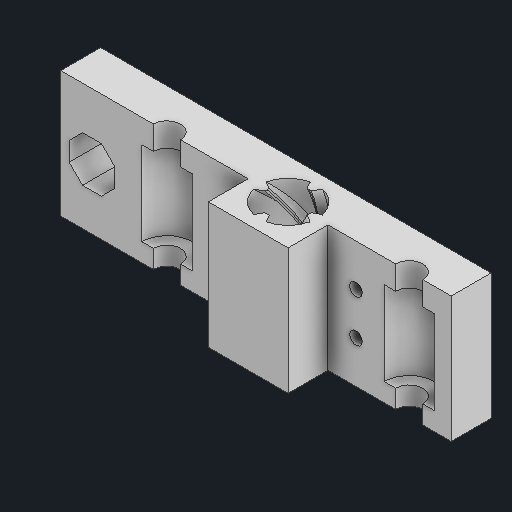
# Autodesk Inventor part: carriage_slider_bottom
Saved by Autodesk Inventor 2025 (Build 290162010, 162A)
## iProperties
Created: 2024-06-23
Part Number: carriage_slider_bottom
Material: Generic
Document SubType Name: Modeling
Designer: mihir
Density: 1 g/cm^3
Appearance: Default
Author: mihir
Autodesk Inventor part; units mm, degrees
ref_plane "YZ Plane" through (0, 0, 0) normal (1, 0, 0) x (0, 1, 0)
ref_plane "XZ Plane" through (0, 0, 0) normal (0, 1, 0) x (-1, 0, 0)
ref_plane "XY Plane" through (0, 0, 0) normal (0, 0, 1) x (1, 0, 0)
sketch "Sketch1" plane through (0, 0, 0) normal (0, 1, 0) x (-1, 0, 0)
  line L0 (-9.5, 9.5) -> (9.5, 9.5)
  line L1 (9.5, 9.5) -> (9.5, -9.5)
  line L2 (9.5, -9.5) -> (-9.5, -9.5)
  line L3 (-9.5, -9.5) -> (-9.5, 9.5)
  line L4 (-9.5, 9.5) -> (9.5, -9.5) construction
  line L5 (9.5, 9.5) -> (-9.5, -9.5) construction
  circle A0 centre (0, 0) radius 6.875
  dimension "d0" = 13.75
  dimension "d1" = 9.5
  constraints: 12 end point, 2 midpoint, 2 parallel, 2 perpendicular, 1 centre point, 1 coincident, 1 horizontal
  measures "d0" diameter of A0
  measures "d1" distance from line of L1 A0.centre
extrude "Extrusion1" add sketch "Sketch1" along normal blind 30
sketch "Sketch2" plane through (0, 30, 0) normal (0, 1, 0) x (1, 0, 0)
  circle A0 centre (0, 0) radius 5 construction
  circle A1 centre (0, 0) radius 6.875 projected
  line L0 (0, -6.875) -> (-1.5825, -6.875)
  line L1 (-1.5825, -6.875) -> (-0.5, -5)
  line L2 (-0.5, -5) -> (0, -5)
  line L3 (0, -6.875) -> (0, -5)
  line L4 (0, -5) -> (0, 0) construction
  line L5 (0, -6.875) -> (1.5825, -6.875)
  line L6 (1.5825, -6.875) -> (0.5, -5)
  line L7 (0.5, -5) -> (0, -5)
  dimension "d4" = 10
  dimension "d5" = 120
  dimension "d6" = 0.5
  constraints: 16 end point, 2 horizontal, 2 symmetric about line, 2 vertical, 2 vertical alignment, 1 coincident, 3 other
  measures "d6" distance of L1.end L2.end
coil "Coil1" sketch "Sketch2" operation add axis through (0, 30, 0) along (0, -1, 0) pitch 40 turns 0.75 hand right contours L1 L2 L3 A1 | A1 L0 L1 | L6 L5 A1 | A1 L3 L7 L6
pattern_circular "Circular Pattern1" count 4 over 360 about axis through (0, 30, 0) along (0, -1, 0) of "Coil1"
sketch "Sketch3" plane through (9.5, 0, -9.5) normal (0, 0, -1) x (-1, 0, 0)
  line L0 (19, 0) -> (19, 30) projected
  line L1 (19, 30) -> (63.65, 30)
  line L2 (63.65, 30) -> (63.65, 0)
  line L3 (63.65, 0) -> (19, 0)
  line L4 (19, 0) -> (19, 30)
  line L5 (0, 0) -> (0, 30) projected
  line L6 (0, 30) -> (-29.35, 30)
  line L7 (-29.35, 30) -> (-29.35, 0)
  line L8 (-29.35, 0) -> (0, 0)
  line L9 (0, 0) -> (0, 30)
  line L10 (19, 0) -> (0, 0) projected
  point P0 (9.5, 0)
  point P1 (0, 0)
  point P2 (19, 0)
  dimension "d18" = 44.65
  dimension "d19" = 29.35
  constraints: 16 end point, 4 parallel, 2 collinear, 2 horizontal, 2 perpendicular
  measures "d18" distance of L2.end L3.end
  measures "d19" distance of L7.end L8.end
extrude "Extrusion2" add sketch "Sketch3" against normal blind 9.5
sketch "Sketch5" plane through (9.5, 0, 0) normal (0, 0, 1) x (1, 0, 0)
  line L0 (13.35, 4.357) -> (19.35, 4.357)
  line L1 (19.35, 4.357) -> (19.35, 24.357)
  line L2 (19.35, 24.357) -> (13.35, 24.357)
  line L3 (13.35, 24.357) -> (13.35, 4.357)
  line L4 (29.35, 0) -> (29.35, 30) projected
  point P0 (-9.5, 0)
  dimension "d22" = 20
  dimension "d23" = 6
  dimension "d24" = 16
  constraints: 8 end point, 2 parallel, 1 horizontal, 1 perpendicular
  measures "d22" distance of L2.end L0.start
  measures "d23" distance of L1.end L2.end
  measures "d24" distance from line of L4 L0.start
revolve "Revolution1" cut sketch "Sketch5" angle 360 about axis through (28.85, 4.357, 0) along (0, 1, 0)
sketch "Sketch6" plane through (9.5, 0, 0) normal (0, 0, 1) x (1, 0, 0)
  line L0 (6.675, 10) -> (6.675, 20) construction
  line L1 (0, 0) -> (0, 30) construction
  line L2 (0, 15) -> (13.35, 15) construction
  line L3 (13.35, 4.357) -> (13.35, 24.357) construction
  point P0 (-9.5, 0)
  point P1 (6.675, 15)
  dimension "d26" = 10
  constraints: 4 end point, 3 midpoint, 1 horizontal, 1 point on line, 1 vertical
  measures "d26" distance of L0.end L0.start
hole "Hole1" at (16.175, 10, 0) at (16.175, 20, 0) direction (0, 0, -1) diameter 3 depth 9.5 tip angle 118
ref_plane "Work Plane1" through (0, 0, 9.5) normal (1, 0, 0) x (0, 0, -1)
mirror "Mirror1" about plane through (0, 0, 9.5) normal (1, 0, 0) of "Revolution1", "Hole1"
sketch "Sketch7" plane through (9.5, 0, 0) normal (0, 0, 1) x (1, 0, 0)
  line L0 (-58.468, 19.789) -> (-53.968, 19.789)
  line L1 (-53.968, 19.789) -> (-50.786, 16.607)
  line L2 (-50.786, 16.607) -> (-50.786, 12.107)
  line L3 (-50.786, 12.107) -> (-53.968, 8.925)
  line L4 (-53.968, 8.925) -> (-58.468, 8.925)
  line L5 (-58.468, 8.925) -> (-61.65, 12.107)
  line L6 (-61.65, 12.107) -> (-61.65, 16.607)
  line L7 (-61.65, 16.607) -> (-58.468, 19.789)
  line L8 (-44.35, 4.357) -> (-44.35, 24.357) construction
  line L9 (-44.35, 14.357) -> (-63.65, 14.357) construction
  line L10 (-63.65, 30) -> (-63.65, 0) construction
  point P0 (-9.5, 0)
  point P1 (-56.218, 14.357)
  dimension "d34" = 2
  dimension "d35" = 4.5
  constraints: 18 end point, 2 point on line, 1 horizontal, 1 midpoint, 1 perpendicular, 17 other
  measures "d34" distance between parallel lines of L10 L6
  measures "d35" distance of L5.end L6.end
extrude "Extrusion3" cut sketch "Sketch7" against normal up to surface (9.5 mm away)
sketch "Sketch8" plane through (38.85, 0, -9.5) normal (0, 0, -1) x (-1, 0, 0)
  line L0 (91, 16.607) -> (91, 12.107) projected
  line L1 (87.818, 19.789) -> (91, 16.607) projected
  line L2 (83.318, 19.789) -> (87.818, 19.789) projected
  line L3 (80.136, 16.607) -> (83.318, 19.789) projected
  line L4 (80.136, 12.107) -> (80.136, 16.607) projected
  line L5 (83.318, 8.925) -> (80.136, 12.107) projected
  line L6 (87.818, 8.925) -> (83.318, 8.925) projected
  line L7 (91, 12.107) -> (87.818, 8.925) projected
  line L8 (91, 12.107) -> (91, 16.607)
  line L9 (87.818, 19.789) -> (83.318, 19.789)
  line L10 (87.818, 19.789) -> (91, 16.607)
  line L11 (83.318, 19.789) -> (80.136, 16.607)
  line L12 (80.136, 16.607) -> (80.136, 12.107)
  line L13 (80.136, 12.107) -> (83.318, 8.925)
  line L14 (87.818, 8.925) -> (91, 12.107)
  line L15 (87.818, 8.925) -> (83.318, 8.925)
  circle A0 centre (85.568, 14.357) radius 4
  circle A1 centre (85.568, 14.357) radius 5.432 construction
  point P0 (38.85, 0)
  dimension "d38" = 8
  constraints: 16 end point, 6 collinear, 3 tangent, 2 centre point, 1 concentric, 1 perpendicular
  measures "d38" diameter of A0
extrude "Extrusion4" add sketch "Sketch8" against normal blind 1
sketch "Sketch9" plane through (0, 0, 0) normal (0, -1, 0) x (1, 0, 0)
  arc A0 (22.85, 0) -> (34.85, 0) centre (28.85, 0) ccw projected
  line L0 (9.5, 0) -> (38.85, 0) projected
  arc A1 (25.6, 0) -> (32.1, 0) centre (28.85, 0) ccw
  line L1 (32.1, 0) -> (25.6, 0)
  point P0 (0, 0)
  point P1 (32.1, 0)
  dimension "d41" = 3.25
  constraints: 2 end point, 2 point on circle, 1 centre point, 1 coincident, 1 collinear, 1 point on line
  measures "d41" radius of A1
extrude "Extrusion5" cut sketch "Sketch9" against normal up to surface (30 mm away) contours L0 A1
mirror "Mirror2" about plane through (0, 0, 9.5) normal (1, 0, 0) of "Extrusion5"
equation "\"d0\" = lead_screw_outer_diameter"
equation "\"d2\" = slider_width"
equation "\"d4\" = lead_screw_diameter"
equation "\"d5\" = screw_profile_angle"
equation "\"d6\" = 0.5 * screw_profile_width"
equation "\"d7\" = screw_pitch"
equation "\"d18\" = slider_length_needle"
equation "\"d19\" = slider_length_back"
equation "\"d20\" = slider_thickness"
equation "\"d22\" = bearing_length"
equation "\"d23\" = 0.5 * bearing_diameter"
equation "\"d26\" = screw_dist"
equation "\"d27\" = screw_diameter"
equation "\"d34\" = octagon_dist"
equation "\"d36\" = slider_thickness"
equation "\"d38\" = needle_hole_diameter"
equation "\"d41\" = 0.5 * rod_free_tolerance + 0.5 * rod_diameter"
equation "\"lead_screw_outer_diameter\" = 13.75"
equation "\"screw_profile_width\" = 1"
equation "\"screw_profile_angle\" = 120deg"
equation "\"screw_pitch\" = 40"
equation "\"slider_width\" = 30"
equation "\"slider_length_needle\" = 44.65"
equation "\"slider_thickness\" = 9.5"
equation "\"bearing_length\" = 20"
equation "\"bearing_diameter\" = 12"
equation "\"screw_diameter\" = 3"
equation "\"bearing_dist\" = 15"
equation "\"slider_length_back\" = 29.35"
equation "\"screw_dist\" = 10"
equation "\"octagon_length\" = 5"
equation "\"octagon_dist\" = 2"
equation "\"needle_hole_diameter\" = 8"
equation "\"rod_diameter\" = 6"
equation "\"rod_free_tolerance\" = 0.5"
equation "\"lead_screw_diameter\" = 10"
body "Solid1"
